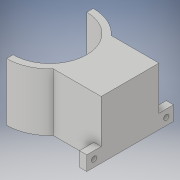
# Autodesk Inventor part: motor support
Saved by Autodesk Inventor 2019 (Build 230136000, 136)
## iProperties
Created: 2023-11-03
Part Number: motor support
Material: Generic
Document SubType Name: Modeling
Designer: ony
Density: 1 g/cm^3
Appearance: Default
Author: ony
Autodesk Inventor part; units mm, degrees
ref_plane "YZ Plane" through (0, 0, 0) normal (1, 0, 0) x (0, 1, 0)
ref_plane "XZ Plane" through (0, 0, 0) normal (0, 1, 0) x (-1, 0, 0)
ref_plane "XY Plane" through (0, 0, 0) normal (0, 0, 1) x (1, 0, 0)
sketch "Sketch1" plane through (0, 0, 0) normal (0, 1, 0) x (-1, 0, 0)
  circle A0 centre (0, 0) radius 32.385
  circle A1 centre (0, 0) radius 38.1
  line L0 (0, 38.1) -> (0, 32.385)
  line L1 (0, -32.385) -> (0, -38.1)
  dimension "d0" = 64.77
  dimension "d1" = 76.2
  constraints: 4 end point, 4 point on circle, 2 centre point, 2 coincident, 2 vertical
  measures "d0" diameter of A0
  measures "d1" diameter of A1
extrude "Extrusion1" add sketch "Sketch1" along normal blind 76.2 contours A0 L1 A1 L0 picked at (-2.826, -35.8766)
sketch "Sketch2" plane through (0, 76.2, 0) normal (0, 1, 0) x (1, 0, 0)
  arc A0 (0, -32.385) -> (0, 32.385) centre (0, 0) ccw projected
  line L0 (32.385, 0) -> (70.485, 0)
  line L1 (70.485, 0) -> (70.485, -25.4)
  line L2 (70.485, -25.4) -> (28.3981, -25.4)
  arc A1 (0, -38.1) -> (0, 38.1) centre (0, 0) ccw projected
  line L3 (70.485, 0) -> (70.485, 25.4)
  line L4 (70.485, 25.4) -> (28.3981, 25.4)
  arc A2 (28.3981, -25.4) -> (28.3981, 25.4) centre (0, 0) ccw
  dimension "d4" = 38.1
  dimension "d5" = 25.4
  dimension "d6" = 25.4
  constraints: 10 end point, 5 point on circle, 2 perpendicular, 1 centre point, 1 horizontal, 1 point on line, 1 vertical
  measures "d4" distance of L0.start L0.end
  measures "d5" distance of L0.end L1.end
  measures "d6" distance of L0.end L3.end
extrude "Extrusion2" add sketch "Sketch2" against normal blind 76.2
sketch "Sketch3" plane through (0, 76.2, 0) normal (0, 1, 0) x (1, 0, 0)
  line L0 (70.485, -25.4) -> (28.3981, -25.4) projected
  line L1 (70.485, -25.4) -> (64.135, -25.4)
  line L2 (64.135, -25.4) -> (64.135, -38.1)
  line L3 (64.135, -38.1) -> (70.485, -38.1)
  line L4 (70.485, -38.1) -> (70.485, -25.4)
  line L5 (28.3981, 25.4) -> (70.485, 25.4) projected
  line L6 (70.485, 25.4) -> (64.135, 25.4)
  line L7 (64.135, 25.4) -> (64.135, 38.1)
  line L8 (64.135, 38.1) -> (70.485, 38.1)
  line L9 (70.485, 38.1) -> (70.485, 25.4)
  point P0 (0, 0)
  dimension "d9" = 6.35
  dimension "d10" = 12.7
  dimension "d11" = 6.35
  dimension "d12" = 12.7
  constraints: 16 end point, 4 parallel, 2 horizontal, 2 perpendicular
  measures "d9" distance of L3.end L2.end
  measures "d10" distance of L2.end L1.end
  measures "d11" distance of L7.end L8.end
  measures "d12" distance of L6.end L7.end
extrude "Extrusion3" add sketch "Sketch3" against normal blind 76.2
sketch "Sketch4" plane through (70.485, 76.2, 38.1) normal (1, 0, 0) x (0, 0, -1)
  line L0 (0, -76.2) -> (0, 0) projected
  line L1 (0, 0) -> (12.7, 0)
  line L2 (12.7, 0) -> (12.7, -76.2)
  line L3 (12.7, -76.2) -> (0, -76.2)
  line L4 (0, -76.2) -> (0, 0)
  line L5 (63.5, 0) -> (63.5, -76.2) projected
  line L6 (76.2, 0) -> (76.2, -76.2) projected
  line L7 (63.5, -76.2) -> (76.2, -76.2)
  line L8 (76.2, -76.2) -> (76.2, 0)
  line L9 (76.2, 0) -> (63.5, 0)
  line L10 (63.5, 0) -> (63.5, -76.2)
  line L11 (0, -76.2) -> (12.7, -76.2)
  line L12 (12.7, -76.2) -> (12.7, -63.5)
  line L13 (12.7, -63.5) -> (0, -63.5)
  line L14 (0, -63.5) -> (0, -76.2)
  line L15 (0, 0) -> (76.2, 0) projected
  line L16 (0, 0) -> (12.7, 0)
  line L17 (12.7, 0) -> (12.7, -12.7)
  line L18 (12.7, -12.7) -> (0, -12.7)
  line L19 (0, -12.7) -> (0, 0)
  line L20 (63.5, -76.2) -> (76.2, -76.2)
  line L21 (76.2, -76.2) -> (76.2, -63.5)
  line L22 (76.2, -63.5) -> (63.5, -63.5)
  line L23 (63.5, -63.5) -> (63.5, -76.2)
  line L24 (63.5, 0) -> (76.2, 0)
  line L25 (76.2, 0) -> (76.2, -12.7)
  line L26 (76.2, -12.7) -> (63.5, -12.7)
  line L27 (63.5, -12.7) -> (63.5, 0)
  point P0 (38.1, -76.2)
  dimension "d15" = 12.7
  dimension "d16" = 12.7
  dimension "d17" = 12.7
  dimension "d18" = 12.7
  dimension "d19" = 12.7
  dimension "d20" = 12.7
  dimension "d21" = 12.7
  dimension "d22" = 12.7
  constraints: 48 end point, 12 parallel, 6 horizontal, 6 perpendicular
  measures "d15" distance of L13.end L12.end
  measures "d16" distance of L12.end L11.end
  measures "d17" distance of L17.end L18.end
  measures "d18" distance of L16.end L17.end
  measures "d19" distance of L22.end L21.end
  measures "d20" distance of L21.end L20.end
  measures "d21" distance of L25.end L26.end
  measures "d22" distance of L24.end L25.end
extrude "Extrusion4" cut sketch "Sketch4" against normal blind 36.5125 contours L0 L18 L2 L13 | L26 L6 L22 L5
sketch "Sketch5" plane through (70.485, 76.2, 38.1) normal (1, 0, 0) x (0, 0, -1)
  line L0 (12.7, -12.7) -> (0, -12.7) projected
  line L1 (0, -76.2) -> (0, 0) projected
  line L2 (12.7, -12.7) -> (0, -12.7)
  line L3 (0, -12.7) -> (0, 0)
  line L4 (0, 0) -> (12.7, 0)
  line L5 (12.7, 0) -> (12.7, -12.7)
  line L6 (76.2, -12.7) -> (63.5, -12.7) projected
  line L7 (63.5, 0) -> (76.2, 0) projected
  line L8 (63.5, -12.7) -> (76.2, -12.7)
  line L9 (76.2, -12.7) -> (76.2, 0)
  line L10 (76.2, 0) -> (63.5, 0)
  line L11 (63.5, 0) -> (63.5, -12.7)
  line L12 (12.7, -63.5) -> (0, -63.5) projected
  line L13 (0, -76.2) -> (12.7, -76.2) projected
  line L14 (12.7, -63.5) -> (0, -63.5)
  line L15 (0, -63.5) -> (0, -76.2)
  line L16 (0, -76.2) -> (12.7, -76.2)
  line L17 (12.7, -76.2) -> (12.7, -63.5)
  line L18 (63.5, -63.5) -> (63.5, -12.7) projected
  line L19 (63.5, -76.2) -> (76.2, -76.2) projected
  line L20 (63.5, -63.5) -> (76.2, -63.5)
  line L21 (76.2, -63.5) -> (76.2, -76.2)
  line L22 (76.2, -76.2) -> (63.5, -76.2)
  line L23 (63.5, -76.2) -> (63.5, -63.5)
  circle A0 centre (6.35, -6.35) radius 2.25
  circle A1 centre (69.85, -6.35) radius 2.25
  circle A2 centre (6.35, -69.85) radius 2.25
  circle A3 centre (69.85, -69.85) radius 2.25
  point P0 (38.1, -76.2)
  dimension "d25" = 4.5
  dimension "d26" = 4.5
  dimension "d27" = 4.5
  dimension "d28" = 4.5
  constraints: 32 end point, 8 parallel, 4 centre point, 4 horizontal, 4 perpendicular
  measures "d25" diameter of A0
  measures "d26" diameter of A1
  measures "d27" diameter of A2
  measures "d28" diameter of A3
extrude "Extrusion5" cut sketch "Sketch5" against normal blind 36.5125 contours A0 | A1 | A2 | A3
thicken "Thicken1" operation add thickness 25.4 both sides no extend neighbours yes toward (0, -1, 0) faces at (53.473, 76.2, 1.3012)
body "Solid1"
